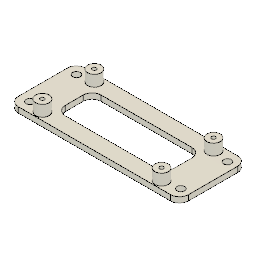
ckt-ledpanel-mount v2.3 (Autodesk Fusion 360 design; units mm, degrees)
Autodesk Fusion 360 part; units mm, degrees
note: some values were not read from the file. Set by a fixed rule: the direction of a hole.
sketch "Sketch1" plane through (0, 0, 0) normal (0, 1, 0) x (1, 0, 0)
  circle A0 centre (14.478, 4.318) radius 3.81
  circle A1 centre (14.478, 33.782) radius 3.81
  circle A2 centre (14.478, 33.782) radius 1.143
  circle A3 centre (91.44, 5.842) radius 2.159
  circle A4 centre (82.042, 4.318) radius 3.81
  circle A5 centre (5.842, 32.258) radius 2.159
  circle A6 centre (14.478, 4.318) radius 1.143
  circle A7 centre (82.042, 33.782) radius 3.81
  circle A8 centre (5.842, 5.842) radius 2.159
  circle A9 centre (82.042, 33.782) radius 1.143
  circle A10 centre (82.042, 4.318) radius 1.143
  circle A11 centre (91.44, 32.258) radius 2.159
  line L0 (5.08, 38.1) -> (91.44, 38.1)
  line L1 (96.52, 33.02) -> (96.52, 5.08)
  line L2 (91.44, 0) -> (5.08, 0)
  line L3 (0, 5.08) -> (0, 33.02)
  arc A12 (5.08, 38.1) -> (0, 33.02) centre (5.08, 33.02) ccw
  arc A13 (0, 5.08) -> (5.08, 0) centre (5.08, 5.08) ccw
  arc A14 (96.52, 33.02) -> (91.44, 38.1) centre (91.44, 33.02) ccw
  arc A15 (91.44, 0) -> (96.52, 5.08) centre (91.44, 5.08) ccw
  line L4 (22.86, 29.21) -> (74.3407, 29.21)
  line L5 (79.4207, 24.13) -> (79.4207, 13.97)
  line L6 (74.3407, 8.89) -> (22.86, 8.89)
  line L7 (17.78, 13.97) -> (17.78, 24.13)
  arc A16 (22.86, 29.21) -> (17.78, 24.13) centre (22.86, 24.13) ccw
  arc A17 (17.78, 13.97) -> (22.86, 8.89) centre (22.86, 13.97) ccw
  arc A18 (74.3407, 8.89) -> (79.4207, 13.97) centre (74.3407, 13.97) ccw
  arc A19 (79.4207, 24.13) -> (74.3407, 29.21) centre (74.3407, 24.13) ccw
  point P0 (0, 38.1)
  point P1 (96.52, 38.1)
  point P2 (96.52, 0)
  point P3 (96.52, 0.0007)
  dimension "d12" = 8.636
  dimension "d13" = 8.636
  dimension "d16" = 67.564
  dimension "d17" = 67.564
  dimension "d18" = 29.464
  dimension "d20" = 96.52
  dimension "d21" = 38.1
  dimension "d22" = 5.08
  dimension "d23" = 5.08
  dimension "d24" = 5.08
  dimension "d25" = 5.08
  dimension "d26" = 5.08
  dimension "d27" = 5.08
  constraint concentric A7 A9
  constraint horizontal L0
  constraint vertical L1
  constraint horizontal L2
  constraint vertical L3
  constraint coincident P0 L3
  constraint coincident P0 L0
  constraint tangent L3 A12
  constraint tangent L0 A12
  constraint concentric A0 A6
  constraint tangent L3 A13
  constraint tangent L2 A13
  constraint concentric A4 A10
  constraint coincident P1 L0
  constraint coincident P1 L1
  constraint tangent L0 A14
  constraint tangent L1 A14
  constraint coincident P2 L2
  constraint coincident P2 L1
  constraint tangent L2 A15
  constraint tangent L1 A15
  constraint horizontal L4
  constraint vertical L5
  constraint horizontal L6
  constraint vertical L7
  constraint tangent L7 A16
  constraint tangent L4 A16
  constraint tangent L7 A17
  constraint tangent L6 A17
  constraint equal A16 A17
  constraint tangent L6 A18
  constraint tangent L5 A18
  constraint equal A16 A18
  constraint tangent L4 A19
  constraint tangent L5 A19
  measures "d12" horizontal distance of A1.centre A5.centre
  measures "d13" horizontal distance of A0.centre A8.centre
  measures "d16" distance of A1.centre A7.centre
  measures "d17" distance of A0.centre A4.centre
  measures "d18" distance of A1.centre A0.centre
  measures "d20" distance of P0 P1
  measures "d21" distance of P1 P2
  measures "d22" radius of A12
  measures "d23" radius of A13
  measures "d24" radius of A14
  measures "d25" radius of A15
  measures "d26" radius of A16
  measures "d27" radius of A19
extrude "Extrude1" add sketch "Sketch1" along normal blind 3.175 contours L0 L1 L2 L3 A12 A13 A14 A15 makes body 1
extrude "Extrude2" add sketch "Sketch1" along normal blind 9.525 separate body contours A0 | A1 | A2 | A4 | A6 | A7 | A9 | A10 makes body 2 at (18.2833, 6.35, -4.1281) makes body 3 at (85.8473, 6.35, -33.5921) makes body 4 at (18.2833, 6.35, -33.5921) makes body 5 at (85.8473, 6.35, -4.1281)
hole "Hole1" at (5.842, 0, -5.842) at (5.842, 0, -32.258) at (91.44, 0, -5.842) at (91.44, 0, -32.258) direction (0, -1, 0) diameter 4.318 depth 2.54 tip angle 118 bodies 1
hole "Hole2" at (14.478, 0, -4.318) at (14.478, 0, -33.782) at (82.042, 0, -33.782) at (82.042, 0, -4.318) direction (0, 1, 0) diameter 2.286 depth 9.525 tip angle 180 bodies 2 3 4 5
